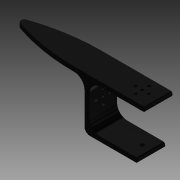
# Autodesk Inventor part: CLAW
Saved by Autodesk Inventor 2014 SP2 (Build 180246200, 246)
## iProperties
Created: 2014-12-14
Part Number: CLAW
Material: Generic
Document SubType Name: Modeling
Designer: Sergei
Density: 1 g/cm^3
Appearance: Glossy - Black
Author: Sergei
Autodesk Inventor part; units mm, degrees
ref_plane "YZ Plane" through (0, 0, 0) normal (1, 0, 0) x (0, 1, 0)
sketch "Sketch1" plane through (0, 0, 0) normal (0, 0, 1) x (1, 0, 0)
  line L0 (0, 0) -> (-53, 0)
  line L1 (-53, 0) -> (-53, 18)
  line L2 (-53, 18) -> (0, 18) construction
  line L3 (-53, 18) -> (-56, 18)
  line L4 (-56, 18) -> (-56, -3)
  line L5 (-56, -3) -> (0, -3)
  line L6 (0, -3) -> (0, 0)
  dimension "d0" = 18
  dimension "d1" = 3
  dimension "d2" = 3
  dimension "d3" = 56
  constraints: 14 end point, 5 perpendicular, 1 coincident, 1 horizontal
  measures "d0" distance between parallel lines of L2 L0
  measures "d1" distance between parallel lines of L4 L1
  measures "d2" distance between parallel lines of L5 L0
  measures "d3" distance between parallel lines of L6 L4
extrude "Extrusion1" add sketch "Sketch1" along normal blind 10
mirror "Mirror1" about plane through (-34.1948, 1.3052, 0) normal (0, 0, -1) of "Extrusion1"
mirror "Mirror2" about plane through (-53, 18, 0) normal (0, 1, 0) of "Extrusion1", "Mirror1"
sketch "Sketch4" plane through (0, -3, -10) normal (0, 0, -1) x (-1, 0, 0)
  line L0 (0, 3) -> (53, 3) projected
  line L1 (0, 0) -> (0, 3) projected
  line L2 (56, 0) -> (0, 0) projected
  line L3 (56, 42) -> (56, 0) projected
  line L4 (56, 42) -> (0, 42) projected
  line L5 (0, 42) -> (0, 39) projected
  line L6 (0, 39) -> (53, 39) projected
  line L7 (53, 39) -> (53, 3) projected
  line L8 (0, 3) -> (53, 3) projected
  line L9 (0, 0) -> (0, 3) projected
  line L10 (56, 0) -> (0, 0) projected
  line L11 (56, 42) -> (56, 0) projected
  line L12 (56, 42) -> (0, 42) projected
  line L13 (0, 42) -> (0, 39) projected
  line L14 (0, 39) -> (53, 39) projected
  line L15 (53, 39) -> (53, 3) projected
extrude "Extrusion4" add sketch "Sketch4" along normal blind 5
mirror "Mirror3" about plane through (0, 0, 0) normal (0, 0, 1) of "Extrusion4"
sketch "Sketch11" plane through (-56, -3, -15) normal (0, -1, 0) x (1, 0, 0)
  line L0 (56, 0) -> (56, 30) projected
  line L1 (56, 30) -> (0, 30) projected
  line L2 (0, 0) -> (0, 30) projected
  line L3 (56, 0) -> (0, 0) projected
  line L4 (56, 0) -> (56, 30) projected
  line L5 (56, 30) -> (0, 30) projected
  line L6 (0, 0) -> (0, 30) projected
  line L7 (56, 0) -> (0, 0) projected
  point P0 (56, 15)
extrude "Extrusion11" cut sketch "Sketch11" against normal blind 10
sketch "Sketch13" plane through (0, 36, -15) normal (1, 0, 0) x (0, 0, -1)
  line L0 (-30, 3) -> (-28, 3)
  line L1 (-28, 3) -> (-28, -29)
  line L2 (-28, -29) -> (-30, -29)
  line L3 (-30, -29) -> (-30, 3)
  line L4 (-30, -29) -> (0, -29) projected
  point P0 (-15, -36)
  dimension "d65" = 2
  constraints: 8 end point, 2 parallel, 1 collinear, 1 horizontal, 1 perpendicular
  measures "d65" distance of L1.end L2.end
extrude "Extrusion13" cut sketch "Sketch13" against normal up to next
mirror "Mirror4" about plane through (0, 0, 0) normal (0, 0, 1) of "Extrusion13"
sketch "Sketch14" plane through (-56, 7, 13) normal (-1, 0, 0) x (0, 0, 1)
  line L0 (-26, 32) -> (-26, 0) projected
  line L1 (-26, 0) -> (0, 0) projected
  line L2 (0, 32) -> (-26, 32) projected
  circle A0 centre (-13, 10) radius 6.5 construction
  line L3 (-13, 10) -> (-26, 10) construction
  line L4 (-13, 10) -> (-13, 32) construction
  circle A1 centre (-13, 10) radius 1.5
  circle A2 centre (-13, 16.5) radius 1.5
  point P0 (-13, -7)
  point P1 (-13, 0)
  dimension "d68" = 13
  dimension "d69" = 22
  dimension "d71" = 3
  dimension "d72" = 3
  constraints: 4 end point, 2 centre point, 2 midpoint, 2 point on line, 2 vertical alignment, 1 coincident, 1 parallel, 1 perpendicular, 2 other
  measures "d69" distance between parallel lines of L2 L3
  measures "d71" diameter of A2
  measures "d72" diameter of A1
extrude "Extrusion14" cut sketch "Sketch14" against normal up to next
pattern_circular "Circular Pattern6" count 4 over 360 about axis through (-56, 17, 0) along (1, 0, 0) of "Extrusion14"
sketch "Sketch15" plane through (-53, 36, 13) normal (0, -1, 0) x (1, 0, 0)
  line L0 (53, -26) -> (53, 0) projected
  line L1 (53, 0) -> (0, 0) projected
  circle A0 centre (37, -13) radius 6.5 construction
  line L2 (37, -13) -> (37, 0) construction
  circle A1 centre (37, -6.5) radius 1.5
  circle A2 centre (37, -13) radius 1.5
  point P0 (53, -13)
  point P1 (53, -13)
  dimension "d78" = 13
  dimension "d79" = 16
  dimension "d80" = 3
  dimension "d81" = 3
  constraints: 3 centre point, 2 coincident, 2 end point, 2 midpoint, 1 horizontal alignment, 1 parallel, 1 perpendicular, 1 point on line
  measures "d78" diameter of A0
  measures "d79" distance between parallel lines of L0 L2
  measures "d80" diameter of A1
  measures "d81" diameter of A2
extrude "Extrusion15" cut sketch "Sketch15" against normal up to next
pattern_circular "Circular Pattern7" count 4 over 360 about axis through (-16, 36, 0) along (0, 1, 0) of "Extrusion15"
sketch "Sketch16" plane through (-56, 7, -15) normal (0, -1, 0) x (1, 0, 0)
  line L0 (0, 2) -> (3, 2) projected
  line L1 (3, 28) -> (3, 2) projected
  line L2 (3, 28) -> (0, 28) projected
  line L3 (0, 2) -> (0, 28) projected
  line L4 (0, 2) -> (3, 2) projected
  line L5 (3, 28) -> (3, 2) projected
  line L6 (3, 28) -> (0, 28) projected
  line L7 (0, 2) -> (0, 28) projected
  point P0 (56, 15)
extrude "Extrusion16" add sketch "Sketch16" along normal blind 14
ref_plane "Work Plane1" through (-47, 34, 13) normal (1, 0, 0) x (0, 0, -1)
sketch "Sketch17" plane through (-47, 34, 13) normal (1, 0, 0) x (0, 0, -1)
  line L0 (0, 0) -> (0, -41) projected
  line L1 (26, -41) -> (0, -41)
  line L2 (0, -41) -> (0, -39)
  line L3 (0, -39) -> (26, -39)
  line L4 (26, -39) -> (26, -41)
  point P0 (13, -34)
  dimension "d92" = 2
  constraints: 8 end point, 2 parallel, 1 horizontal, 1 perpendicular, 1 point on line
  measures "d92" distance of L1.end L2.end
extrude "Extrusion17" add sketch "Sketch17" along normal blind 40
ref_plane "Work Plane3" through (-47, -5, 13) normal (0, 1, 0) x (1, 0, 0)
sketch "Sketch18" plane through (-47, -5, 13) normal (0, 1, 0) x (1, 0, 0)
  circle A0 centre (31, 13) radius 1.5 projected
  circle A1 centre (31, 13) radius 2
  point P0 (47, 13)
  dimension "d95" = 4
  constraints: 1 centre point, 1 coincident
  measures "d95" diameter of A1
extrude "Extrusion18" cut sketch "Sketch18" against normal up to next contours A0 | A1
sketch "Sketch23" plane through (0, 36, 13) normal (0, 0, 1) x (1, 0, 0)
  line L0 (0, 0) -> (-53, 0) projected
  line L1 (-56, 3) -> (0, 3) projected
  line L2 (-56, -43) -> (-56, 3) projected
  line L3 (-7, -43) -> (-56, -43) projected
  line L4 (-47, -41) -> (-7, -41) projected
  line L5 (-53, 0) -> (-53, -43) projected
  line L6 (0, 0) -> (-53, 0) projected
  line L7 (0, 3) -> (0, 0) projected
  line L8 (-56, 3) -> (0, 3) projected
  line L9 (-56, -43) -> (-56, 3) projected
  line L10 (-53, -43) -> (-56, -43) projected
  line L11 (0, 0) -> (-56, 0)
  line L12 (-56, 0) -> (-56, 4.5)
  line L13 (-56, 4.5) -> (0, 4.5)
  line L14 (0, 4.5) -> (0, 0)
  line L15 (-7, -41) -> (-56, -41)
  line L16 (-56, -41) -> (-56, -45.5)
  line L17 (-56, -45.5) -> (-7, -45.5)
  line L18 (-7, -45.5) -> (-7, -41)
  point P0 (0, -36)
  dimension "d110" = 3
  dimension "d111" = 2
  dimension "d112" = 1.5
  dimension "d113" = 2.5
  constraints: 16 end point, 4 parallel, 2 horizontal, 2 perpendicular, 1 collinear, 1 point on line
  measures "d110" distance between parallel lines of L0 L1
  measures "d111" distance between parallel lines of L3 L4
  measures "d112" distance between parallel lines of L1 L13
  measures "d113" distance between parallel lines of L17 L3
sketch "Sketch24" plane through (-56, 39, 13) normal (0, 1, 0) x (1, 0, 0)
  circle A0 centre (40, 19.5) radius 1.5 projected
  circle A1 centre (46.5, 13) radius 1.5 projected
  circle A2 centre (33.5, 13) radius 1.5 projected
  circle A3 centre (40, 6.5) radius 1.5 projected
  circle A4 centre (40, 13) radius 1.5 projected
  line L0 (56, 26) -> (0, 26) projected
  line L1 (0, 0) -> (0, 26) projected
  line L2 (0, 0) -> (56, 0) projected
  line L3 (56, 0) -> (56, 26) projected
  point P0 (56, 13)
  dimension "d114" = 26
  measures "d114" distance between parallel lines of L2 L0
extrude "Extrusion22" add sketch "Sketch23" against normal up to surface (26 mm away) contours L0 L11 L2 L1 L7 | L1 L12 L13 L14 | L15 L4 L18 L3 L5 | L5 L3 L2 L15 | L3 L18 L17 L16
sketch "Sketch25" plane through (-53, 36, 13) normal (0, 0, 1) x (1, 0, 0)
  line L0 (-3, 4.5) -> (-3, -45.5) projected
  line L1 (-3, -45.5) -> (46, -45.5) projected
  line L2 (46, -41) -> (46, -45.5) projected
  line L3 (46, -41) -> (0, -41) projected
  line L4 (0, 0) -> (0, -41) projected
  line L5 (53, 0) -> (0, 0) projected
  line L6 (53, 4.5) -> (53, 0) projected
  line L7 (53, 4.5) -> (-3, 4.5) projected
  point P0 (53, -36)
  dimension "d117" = 3
  measures "d117" distance between parallel lines of L4 L0
sketch "Sketch26" plane through (-56, -9.5, -13) normal (-1, 0, 0) x (0, 0, 1)
  line L0 (0, 0) -> (0, 50) projected
  line L1 (26, 0) -> (0, 0) projected
  line L2 (26, 50) -> (26, 0) projected
  line L3 (26, 50) -> (0, 50) projected
  circle A0 centre (13, 20) radius 1.5 projected
  circle A1 centre (19.5, 26.5) radius 1.5 projected
  circle A2 centre (6.5, 26.5) radius 1.5 projected
  circle A3 centre (13, 26.5) radius 1.5 projected
  circle A4 centre (13, 33) radius 1.5 projected
  line L4 (0, 0) -> (0, 50) projected
  line L5 (26, 0) -> (0, 0) projected
  line L6 (26, 50) -> (26, 0) projected
  circle A5 centre (13, 20) radius 1.5 projected
  circle A6 centre (19.5, 26.5) radius 1.5 projected
  circle A7 centre (6.5, 26.5) radius 1.5 projected
  circle A8 centre (13, 26.5) radius 1.5 projected
  circle A9 centre (13, 33) radius 1.5 projected
  line L7 (26, 50) -> (0, 50) projected
  point P0 (13, 9.5)
extrude "Extrusion23" add sketch "Sketch26" along normal blind 2
sketch "Sketch27" plane through (0, 40.5, 13) normal (0, 1, 0) x (1, 0, 0)
  line L0 (-58, 26) -> (0, 26) projected
  line L1 (0, 0) -> (0, 26) projected
  circle A0 centre (-16, 13) radius 6.5 construction
  circle A1 centre (-16, 19.5) radius 1.5
  circle A2 centre (-16, 13) radius 1.5
  line L2 (-16, 13) -> (0, 13) construction
  line L3 (-16, 13) -> (-16, 26) construction
  dimension "d121" = 13
  dimension "d120" = 3
  dimension "d122" = 3
  dimension "d123" = 16
  constraints: 4 end point, 2 centre point, 1 coincident, 1 midpoint, 1 perpendicular, 1 point on line, 1 vertical, 1 vertical alignment, 2 other
  measures "d120" diameter of A1
  measures "d122" diameter of A2
  measures "d123" distance between parallel lines of L1 L3
extrude "Extrusion24" cut sketch "Sketch27" against normal up to surface (4.5 mm away)
pattern_circular "Circular Pattern8" count 4 over 360 about axis through (-16, 40.5, 0) along (0, -1, 0) of "Extrusion24"
sketch "Sketch28" plane through (-53, -5, 13) normal (0, 1, 0) x (1, 0, 0)
  circle A0 centre (37, 13) radius 1.5 projected
  circle A1 centre (37, 13) radius 2
  point P0 (53, 13)
  dimension "d129" = 4
  constraints: 1 centre point, 1 coincident
  measures "d129" diameter of A1
extrude "Extrusion25" cut sketch "Sketch28" against normal up to next contours A0 | A1
sketch "Sketch29" plane through (-58, -9.5, -13) normal (-1, 0, 0) x (0, 0, 1)
  line L0 (0, 50) -> (0, 0) projected
  line L1 (26, 0) -> (26, 50) projected
  line L2 (26, 50) -> (0, 50) projected
  line L3 (26, 45.5) -> (0, 45.5) projected
  point P0 (13, 9.5)
extrude "Extrusion26" add sketch "Sketch29" along normal blind 79.25
sketch "Sketch30" plane through (0, 40.5, 13) normal (0, 1, 0) x (1, 0, 0)
  line L0 (-137.25, 26) -> (0, 26) projected
  line L1 (-137.25, 0) -> (-137.25, 26) projected
  line L2 (0, 0) -> (-137.25, 0) projected
  arc A0 (-137.25, 13) -> (-68.625, 0) centre (-68.625, 187.6304) ccw
  arc A1 (-68.625, 26) -> (-137.25, 13) centre (-68.625, -161.6304) ccw
  point P0 (0, 13)
  constraints: 4 point on circle, 3 midpoint, 2 centre point, 2 tangent
extrude "Extrusion27" cut sketch "Sketch30" against normal up to next
fillet "Fillet9" radius 3 1 edges at (-137.25, 38.25, 0)
fillet "Fillet10" radius 10 1 edges at (-58, 36, 0)
fillet "Fillet11" radius 10 1 edges at (-53, 36, 0)
fillet "Fillet12" radius 5 1 edges at (-58, -9.5, 0)
fillet "Fillet13" radius 2 4 edges at (0, 40.5, 0) (0, 36, 0) (-7, -9.5, 0) (-7, -5, 0)
fillet "Fillet14" radius 10 1 edges at (-53, -5, 0)
equation "\"d72\" = d71"
body "Solid1"
